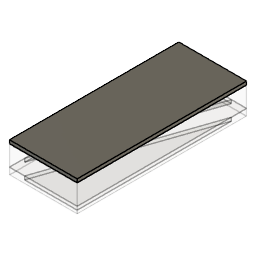
V4.1 (Autodesk Fusion 360 design; units mm, degrees)
part number: 2026-06-09-16-16-10-076
part number: 2026-06-09-16-22-03-425
part number: 2026-06-09-16-27-02-726
part number: 2026-06-09-16-31-41-976
part number: 2026-06-09-16-59-11-533
part number: 2026-06-09-17-00-24-475
Autodesk Fusion 360 part; units mm, degrees
sketch "Esquisse1" plane through (0, 0, 0) normal (0, 0, 1) x (1, 0, 0)
  line L0 (0, 0) -> (20, 0)
  line L1 (20, 0) -> (20, 50)
  line L2 (20, 50) -> (0, 50)
  line L3 (0, 50) -> (0, 0)
  dimension "d5" = 20
  dimension "d6" = 50
  constraint horizontal L0
  constraint vertical L1
  constraint horizontal L2
  constraint vertical L3
  constraint coincident L0.start L3.end
  measures "d5" distance of L0.start L0.end
  measures "d6" distance of L0.start L2.end
extrude "Extrusion1" add sketch "Esquisse1" along normal blind 1 makes body 1 in component "support"
sketch "Esquisse1 (2)" plane through (0, 0, 1) normal (0, 0, 1) x (-1, 0, 0) in component "plaque_bas_droite"
  line L0 (0, -50) -> (0, 0)
  line L1 (0, 0) -> (-20, 0)
  line L2 (-20, 0) -> (-20, -50)
  line L3 (-20, -50) -> (0, -50)
  spline S0 degree 5 poles (-4.5, 0) (-5.12, -1.82) (-6.36, -5.46) (-8.22, -10.92) (-10.7, -18.2) (-13.8, -27.3) (-16.28, -34.58) (-18.14, -40.04) (-19.38, -43.68) (-20, -45.5) knots 0 0 0 0 0 0 0.2 0.4 0.6 0.8 1 1 1 1 1 1
  dimension "d10" = 4.5
  dimension "d11" = 4.5
  constraint coincident L1 S0.start
  constraint coincident L2 S0.end
  measures "d10" distance of L2.end S0.end
  measures "d11" distance of L0.end S0.start
extrude "Extrusion1'" add sketch "Esquisse1 (2)" along normal blind 1 separate body contours L1 L2 S0 makes body 2 in component "plaque_bas_droite"
sketch "Esquisse1 (3)" plane through (0, 0, 1) normal (0, 0, 1) x (-1, 0, 0) in component "plaque_haut_gauche"
  line L0 (0, -50) -> (0, 0)
  line L1 (0, 0) -> (-20, 0)
  line L2 (-20, 0) -> (-20, -50)
  line L3 (-20, -50) -> (0, -50)
  spline S0 degree 5 poles (0, -4.5) (-0.62, -6.32) (-1.86, -9.96) (-3.72, -15.42) (-6.2, -22.7) (-9.3, -31.8) (-11.78, -39.08) (-13.64, -44.54) (-14.88, -48.18) (-15.5, -50) knots 0 0 0 0 0 0 0.2 0.4 0.6 0.8 1 1 1 1 1 1
  dimension "d15" = 4.5
  dimension "d16" = 4.5
  constraint coincident L0 S0.start
  constraint coincident L3 S0.end
  measures "d15" distance of L2.end S0.end
  measures "d16" distance of L0.end S0.start
extrude "Extrusion1''" add sketch "Esquisse1 (3)" along normal blind 1 separate body contours L0 L3 S0 makes body 3 in component "plaque_haut_gauche"
extrude "Extrusion2" add 1 faces at (6.6667, 33.3333, 1) along direction (0, 0, 1) blind 1 on bodies 1 bodies 1 in component "support"
copy_body "CopierCollerCorps1" bodies 3 2 makes body 4 makes body 5 in component "support"
combine "Combiner1" operation cut target body 1 tool bodies 4 5 in component "support"
extrude "Extrusion1'''" add 1 faces at (5.1667, 34.8333, 2) along direction (0, 0, 1) blind 6 separate body on bodies 3 makes body 6 in component "mousse"
extrude "Extrusion2'" add 1 faces at (14.8333, 15.1667, 2) along direction (0, 0, 1) blind 6 separate body on bodies 2 makes body 7 in component "mousse"
extrude "Extrusion3" add 1 faces at (11.8333, 33.3333, 2) along direction (0, 0, 1) blind 6 on bodies 1 bodies 6 7 in component "mousse"
extrude "Extrusion1''''" add 1 faces at (6.6667, 33.3333, 8) along direction (0, 0, 1) blind 1 separate body on bodies 6 makes body 8 in component "plateau"
component "support" placed x (1, 0, 0) y (0, 1, 0) z (0, 0, 1) at (0, 0, 0)
component "plaque_bas_droite" placed x (1, 0, 0) y (0, 1, 0) z (0, 0, 1) at (0, 0, 0)
component "plaque_haut_gauche" placed x (1, 0, 0) y (0, 1, 0) z (0, 0, 1) at (0, 0, 0)
component "mousse" placed x (1, 0, 0) y (0, 1, 0) z (0, 0, 1) at (0, 0, 0)
component "plateau" placed x (1, 0, 0) y (0, 1, 0) z (0, 0, 1) at (0, 0, 0)
equation "largeur = 20 mm"
equation "longeur = 50 mm"
equation "ecart_au_carré = 9 mm"
equation "ecart_coté = ( ecart_au_carré / 2 )"
equation "d5 = largeur"
equation "d6 = longeur"
equation "Hauteur_support = 1 mm"
equation "d8 = Hauteur_support"
equation "d10 = ecart_coté"
equation "d11 = ecart_coté"
equation "epaisseur = 1 mm"
equation "d15 = ecart_coté"
equation "d16 = ecart_coté"
equation "d17 = epaisseur"
equation "d19 = epaisseur"
equation "mousse = 6 mm"
equation "d22 = mousse"
equation "d24 = mousse"
equation "d26 = mousse"
equation "d28 = epaisseur"
